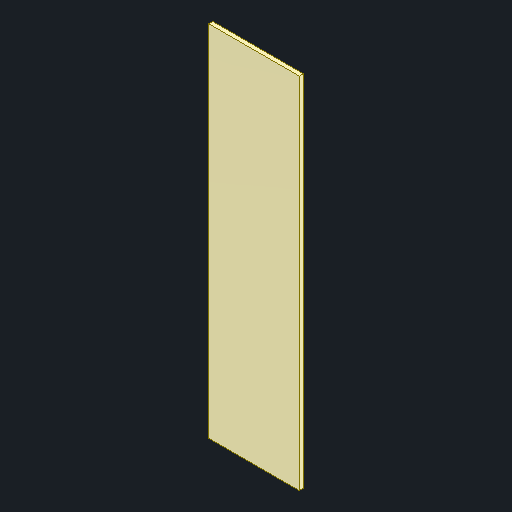
# Autodesk Inventor part: back
Saved by Autodesk Inventor 2023 (Build 270158000, 158)
## iProperties
Created: 2024-04-30
Part Number: back
Material: Nylon 6/6
Document SubType Name: Modeling
Designer: szymo
Density: 1.13 g/cm^3
Appearance: Nylon 6
Mass: 18.1026 g
Surface Area: 169.12 cm^2
Volume: 16.02 cm^3
Author: szymo
Autodesk Inventor part; units mm, degrees
ref_plane "YZ Plane" through (0, 0, 0) normal (1, 0, 0) x (0, 1, 0)
ref_plane "XZ Plane" through (0, 0, 0) normal (0, 1, 0) x (-1, 0, 0)
ref_plane "XY Plane" through (0, 0, 0) normal (0, 0, 1) x (1, 0, 0)
ref_plane "Work Plane1" through (0, 0, 0) normal (0, 0, 1) x (1, 0, 0)
sketch "Sketch1" plane through (0, 0, 0) normal (0, 0, 1) x (1, 0, 0)
  line L0 (0, 0) -> (0, 68)
  line L1 (0, 68) -> (-3.5, 68)
  line L2 (-3.5, 0) -> (-3.5, 68)
  line L3 (0, 0) -> (-3.5, 0)
  line L4 (-3.5, 7) -> (-3.5, 0)
  line L5 (-3.5, 7) -> (-33.5, 7)
  line L6 (-33.5, 7) -> (-33.5, 0)
  line L7 (-6.5, 0) -> (-33.5, 0)
  line L8 (-3.5, 0) -> (-6.5, 0)
  line L9 (-33.5, 19) -> (-33.5, 24)
  line L10 (-33.5, 19) -> (-3.5, 19)
  line L11 (-3.5, 19) -> (-3.5, 24)
  line L12 (-3.5, 24) -> (-33.5, 24)
  line L13 (-33.5, 49) -> (-33.5, 44)
  line L14 (-3.5, 44) -> (-33.5, 44)
  line L15 (-3.5, 49) -> (-3.5, 44)
  line L16 (-33.5, 49) -> (-3.5, 49)
  line L17 (-3.5, 61) -> (-3.5, 68)
  line L18 (-3.5, 68) -> (-6.5, 68)
  line L19 (-6.5, 68) -> (-33.5, 68)
  line L20 (-33.5, 61) -> (-33.5, 68)
  line L21 (-3.5, 61) -> (-33.5, 61)
  line L22 (-34.5, 123) -> (10.5, 123)
  line L23 (10.5, -55) -> (-34.5, -55)
  line L24 (10.5, -55) -> (10.5, 123)
  line L25 (-34.5, 123) -> (-34.5, -55)
  circle A0 centre (-30.5, 64.5) radius 2.3
  circle A1 centre (-11.8324, 64.5) radius 2.3
  circle A2 centre (-18.5, 21.5) radius 2.3
  circle A3 centre (-18.5, 46.5) radius 2.3
extrude "Extrusion1" add sketch "Sketch1" along normal blind 2 contours L3 L2 L1 L0 | L8 L7 L6 L5 L2 | L2 L21 L20 L19 L18 | L10 L9 L12 L2 | L2 L14 L13 L16 | L22 L24 L23 L25 | A0 | A1 | A2 | A3
body "Solid1"
